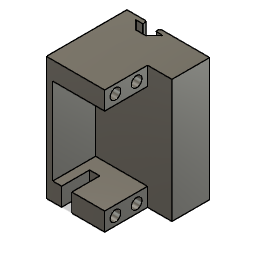
Servo Mount v5 (Autodesk Fusion 360 design; units mm, degrees)
Autodesk Fusion 360 part; units mm, degrees
sketch "Sketch1" plane through (0, 0, 0) normal (0, 0, 1) x (1, 0, 0)
  line L0 (-21, 58) -> (21, 58)
  line L1 (21, 58) -> (21, 0)
  line L2 (21, 0) -> (-21, 0)
  line L3 (-21, 0) -> (-21, 58)
  dimension "d1" = 42
  dimension "d2" = 58
  constraint horizontal L0
  constraint vertical L1
  constraint horizontal L2
  constraint vertical L3
  constraint midpoint origin L2
  measures "d1" distance of L0.start L0.end
  measures "d2" distance of L0.start L2.end
extrude "Extrude1" add sketch "Sketch1" along normal blind 38 makes body 1
sketch "Sketch2" plane through (0, 0, 38) normal (0, 0, 1) x (1, 0, 0)
  line L0 (-21, 0) -> (21, 0)
  line L1 (21, 0) -> (21, 58)
  line L2 (21, 58) -> (-21, 58)
  line L3 (-21, 58) -> (-21, 0)
  line L4 (21, 58) -> (-21, 58)
  line L5 (-21, 58) -> (-21, 0)
  line L6 (-21, 0) -> (21, 0)
  line L7 (21, 0) -> (21, 58)
  line L8 (4, 58) -> (4, 0)
  line L9 (4, 49.4) -> (-18, 49.4)
  line L10 (-18, 49.4) -> (-18, 8.6)
  line L11 (-18, 8.6) -> (4, 8.6)
  line L12 (4, 8.6) -> (4, 49.4)
  line L13 (-18, 49.4) -> (-18, 58) construction
  line L14 (-18, 8.6) -> (-18, 0) construction
  line L15 (-13.8, 8.6) -> (-13.8, 0)
  line L16 (-9, 8.6) -> (-9, 0)
  dimension "d5" = 25
  dimension "d7" = 40.8
  dimension "d8" = 4.2
  dimension "d9" = 4.8
  constraint horizontal L4
  constraint vertical L5
  constraint horizontal L6
  constraint vertical L7
  constraint coincident L0.start L3.end
  constraint coincident L1.end L2.start
  constraint coincident L4 L8.start
  constraint coincident L6 L8.end
  constraint perpendicular L6 L8
  constraint horizontal L9
  constraint vertical L10
  constraint horizontal L11
  constraint vertical L12
  constraint coincident L8 L9.start
  constraint coincident L2 L13.end
  constraint perpendicular L2 L13
  constraint coincident L6 L14.end
  constraint perpendicular L6 L14
  constraint equal L13 L14
  constraint coincident L11 L15.start
  constraint coincident L0 L15.end
  constraint perpendicular L0 L15
  constraint coincident L11 L16.start
  constraint coincident L6 L16.end
  constraint perpendicular L6 L16
  measures "d5" distance of L5 L8
  measures "d7" distance of L9.end L10.end
  measures "d8" distance of L14 L15
  measures "d9" distance of L15 L16
extrude "Extrude2" cut sketch "Sketch2" against normal blind 20.2 contours L8 L9 L10 L11 L12 | L0 L1 L2 L4 L6 L7 L8 L12 bodies 1
extrude "Extrude3" cut sketch "Sketch2" against normal blind 13.2 contours L0 L6 L11 L15 L16 bodies 1
sketch "Sketch3" plane through (0, 58, 0) normal (0, 1, 0) x (-1, 0, 0)
  line L0 (-4, 38) -> (-4, 17.8)
  line L1 (-4, 17.8) -> (-21, 17.8)
  line L2 (-21, 17.8) -> (-21, 0)
  line L3 (-21, 0) -> (21, 0)
  line L4 (21, 0) -> (21, 38)
  line L5 (21, 38) -> (-4, 38)
  line L6 (-21, 0) -> (-18, 0)
  line L7 (-18, 0) -> (-18, 17.8)
  line L8 (-18, 17.8) -> (-21, 17.8)
  line L9 (-21, 17.8) -> (-21, 0)
  dimension "d14" = 3
  constraint horizontal L6
  constraint vertical L7
  constraint horizontal L8
  constraint vertical L9
  constraint coincident L1 L7.end
  constraint coincident L2.end L3.start
  measures "d14" distance of L2.end L6.end
extrude "Extrude4" cut sketch "Sketch3" against normal blind 65 contours L1 L2 L3 L6 L7 L8 L9 bodies 1
sketch "Sketch4" plane through (4, 0, 0) normal (1, 0, 0) x (0, 0, -1)
  line L0 (-38, 58) -> (-38, 49.4)
  line L1 (-38, 49.4) -> (-17.8, 49.4)
  line L2 (-17.8, 49.4) -> (-17.8, 58)
  line L3 (-17.8, 58) -> (-38, 58)
  line L4 (-38, 58) -> (-17.8, 58) construction
  line L5 (-17.8, 58) -> (-17.8, 49.4) construction
  line L6 (-17.8, 49.4) -> (-38, 49.4) construction
  line L7 (-38, 49.4) -> (-38, 58) construction
  line L8 (-27.9, 58) -> (-27.9, 49.4) construction
  line L9 (-38, 53.9) -> (-17.8, 53.9) construction
  line L10 (-32.9, 53.9) -> (-22.9, 53.9)
  circle A0 centre (-32.9, 53.9) radius 2.5
  circle A1 centre (-22.9, 53.9) radius 2.5
  circle A2 centre (-22.9, 4.1) radius 2.5
  line L11 (-22.9, 4.1) -> (-32.9, 4.1) construction
  line L12 (-38, 0) -> (-17.8, 0)
  line L13 (-38, 0) -> (-38, 8.6)
  circle A3 centre (-32.9, 4.1) radius 2.5
  line L14 (-17.8, 0) -> (-38, 0) construction
  line L15 (-17.8, 8.6) -> (-17.8, 0) construction
  line L16 (-27.9, 0) -> (-27.9, 8.6) construction
  line L17 (-17.8, 4.1) -> (-38, 4.1) construction
  line L18 (-17.8, 0) -> (-17.8, 8.6)
  line L19 (-38, 8.6) -> (-38, 0) construction
  line L20 (-17.8, 8.6) -> (-38, 8.6)
  line L21 (-38, 8.6) -> (-17.8, 8.6) construction
  point P0 (-27.9, 53.9)
  point P1 (-27.9, 4.1)
  dimension "d17" = 4.5
  dimension "d18" = 10
  dimension "d19" = 5
  dimension "d20" = 5
  dimension "d21" = 4.5
  dimension "d22" = 10
  dimension "d23" = 5
  dimension "d24" = 5
  constraint horizontal L4
  constraint vertical L5
  constraint horizontal L6
  constraint vertical L7
  constraint coincident L1.end L2.start
  constraint coincident L0.start L3.end
  constraint midpoint L4 L8.start
  constraint midpoint L6 L8.end
  constraint coincident L7 L9.start
  constraint coincident L5 L9.end
  constraint perpendicular L5 L9
  constraint midpoint L9 P0
  constraint coincident L9 L10.start
  constraint coincident L9 L10.end
  constraint parallel L9 L10
  constraint midpoint P0 L10
  constraint coincident L10.start A0.centre
  constraint coincident L10.end A1.centre
  constraint coincident L13.end L19.start
  constraint coincident L12.end L14.start
  constraint midpoint L16.start L14
  constraint midpoint L16.end L21
  constraint coincident L17.start L15
  constraint coincident L17.end L13
  constraint perpendicular L13 L17
  constraint midpoint P1 L17
  constraint coincident A2.centre L17
  constraint coincident L11.end L17
  constraint parallel L11 L17
  constraint midpoint P1 L11
  constraint coincident A2.centre L11.start
  constraint coincident L11.end A3.centre
  measures "d17" distance of L6 L9
  measures "d18" distance of L10.start L10.end
  measures "d19" diameter of A0
  measures "d20" diameter of A1
  measures "d21" distance of L17 L21
  measures "d22" distance of L11.end A2.centre
  measures "d23" diameter of A2
  measures "d24" diameter of A3
extrude "Extrude5" cut sketch "Sketch4" against normal blind 6 contours A0 | A1 | A2 | A3 bodies 1
sketch "profile" plane through (0, 0, 0) normal (0, 1, 0) x (1, 0, 0) in component "20 mm x 20 mm T-Slot v1"
  circle A0 centre (0, 0) radius 2.5
  line L0 (0, -3.9) -> (-2.5, -3.9)
  line L1 (4, -4) -> (-4, 4) construction
  line L2 (-3.9092, -3.9092) -> (4, 4) construction
  line L3 (10, -10) -> (-10, -10) construction
  line L4 (-10, -10) -> (-10, 10) construction
  line L5 (-10, 10) -> (10, 10) construction
  line L6 (10, 10) -> (10, -10) construction
  line L7 (10, -10) -> (-10, 10) construction
  line L8 (-10, -10) -> (10, 10) construction
  line L9 (8, -8) -> (-8, -8) construction
  line L10 (-8, -8) -> (-8, 8) construction
  line L11 (-8, 8) -> (8, 8) construction
  line L12 (8, 8) -> (8, -8) construction
  line L13 (8, -8) -> (-8, 8) construction
  line L14 (-8, -8) -> (8, 8) construction
  line L15 (0, -8) -> (0, -10) construction
  line L16 (0, -9) -> (-3.1, -9) construction
  line L17 (-3.1, -8) -> (-3.1, -9.6)
  line L18 (-1.75, -10) -> (-1.75, -9.6) construction
  line L19 (0, -9.6) -> (-3.5, -9.6) construction
  line L20 (-3.1, -9.6) -> (-3.5, -9.6)
  line L21 (-3.5, -9.6) -> (-3.5, -10)
  line L22 (0, 0) -> (0, -8) construction
  line L23 (-3.5, -10) -> (-10, -10)
  line L24 (-3.9092, -3.9092) -> (-2.5, -3.9) construction
  line L25 (-8, -8) -> (-6.6, -8) construction
  line L26 (-8, -8) -> (-8, -7) construction
  line L27 (-2.5, -3.9) -> (-6.6, -8)
  line L28 (-6.6, -8) -> (-3.1, -8)
  line L29 (0, -2.5) -> (0, -3.9) construction
  line L30 (-3.9, 0) -> (-3.9, -2.5)
  line L31 (-3.9, -2.5) -> (-8, -6.6)
  line L32 (-8, -6.6) -> (-8, -3.1)
  line L33 (-8, -3.1) -> (-9.6, -3.1)
  line L34 (-9.6, -3.1) -> (-9.6, -3.5)
  line L35 (-9.6, -3.5) -> (-10, -3.5)
  line L36 (-10, -3.5) -> (-10, -10)
  line L37 (0, 0) -> (10, 0) construction
  line L38 (3.9, 0) -> (3.9, -2.5)
  line L39 (3.9, -2.5) -> (8, -6.6)
  line L40 (8, -6.6) -> (8, -3.1)
  line L41 (8, -3.1) -> (9.6, -3.1)
  line L42 (9.6, -3.1) -> (9.6, -3.5)
  line L43 (9.6, -3.5) -> (10, -3.5)
  line L44 (10, -3.5) -> (10, -10)
  line L45 (0, -3.9) -> (2.5, -3.9)
  line L46 (6.6, -8) -> (3.1, -8)
  line L47 (3.1, -8) -> (3.1, -9.6)
  line L48 (3.1, -9.6) -> (3.5, -9.6)
  line L49 (3.5, -9.6) -> (3.5, -10)
  line L50 (3.5, -10) -> (10, -10)
  line L51 (2.5, -3.9) -> (6.6, -8)
  line L52 (-3.9, 0) -> (-3.9, 2.5)
  line L53 (-3.9, 2.5) -> (-8, 6.6)
  line L54 (-8, 6.6) -> (-8, 3.1)
  line L55 (-8, 3.1) -> (-9.6, 3.1)
  line L56 (-9.6, 3.1) -> (-9.6, 3.5)
  line L57 (-9.6, 3.5) -> (-10, 3.5)
  line L58 (-10, 3.5) -> (-10, 10)
  line L59 (0, 3.9) -> (-2.5, 3.9)
  line L60 (-6.6, 8) -> (-3.1, 8)
  line L61 (-3.1, 8) -> (-3.1, 9.6)
  line L62 (-3.1, 9.6) -> (-3.5, 9.6)
  line L63 (-3.5, 9.6) -> (-3.5, 10)
  line L64 (-3.5, 10) -> (-10, 10)
  line L65 (-2.5, 3.9) -> (-6.6, 8)
  line L66 (0, 3.9) -> (2.5, 3.9)
  line L67 (6.6, 8) -> (3.1, 8)
  line L68 (3.1, 8) -> (3.1, 9.6)
  line L69 (3.1, 9.6) -> (3.5, 9.6)
  line L70 (3.5, 9.6) -> (3.5, 10)
  line L71 (3.5, 10) -> (10, 10)
  line L72 (2.5, 3.9) -> (6.6, 8)
  line L73 (3.9, 0) -> (3.9, 2.5)
  line L74 (8, 6.6) -> (8, 3.1)
  line L75 (8, 3.1) -> (9.6, 3.1)
  line L76 (9.6, 3.1) -> (9.6, 3.5)
  line L77 (9.6, 3.5) -> (10, 3.5)
  line L78 (10, 3.5) -> (10, 10)
  line L79 (3.9, 2.5) -> (8, 6.6)
  dimension "d3_1" = 5
  dimension "d7_1" = 8
  dimension "d8_1" = 8
  dimension "d9_1" = 20
  dimension "d10_1" = 20
  dimension "d11_1" = 16
  dimension "d12_1" = 16
  dimension "d13_1" = 3.1
  dimension "d14_1" = 0.4
  dimension "d15_1" = 3.5
  dimension "d20_1" = 2.5
  dimension "d21_1" = 1.4
  constraint coincident A0.centre L22.start
  constraint horizontal L0
  constraint coincident L1 A0.centre
  constraint coincident L2 A0.centre
  constraint horizontal L3
  constraint perpendicular L3 L4
  constraint parallel L3 L5
  constraint parallel L4 L6
  constraint coincident L7 A0.centre
  constraint coincident L8 A0.centre
  constraint horizontal L9
  constraint perpendicular L9 L10
  constraint parallel L9 L11
  constraint parallel L10 L12
  constraint coincident L13 A0.centre
  constraint coincident L14 A0.centre
  constraint midpoint L9 L15.start
  constraint midpoint L3 L15.end
  constraint midpoint L15 L16.start
  constraint perpendicular L15 L16
  constraint coincident L9 L17.start
  constraint perpendicular L3 L17
  constraint coincident L16.end L17
  constraint vertical L18
  constraint coincident L3 L18.start
  constraint coincident L15 L19.start
  constraint perpendicular L15 L19
  constraint coincident L18.end L19
  constraint coincident L19 L17.end
  constraint coincident L3 L21.end
  constraint perpendicular L3 L21
  constraint midpoint L18.end L19
  constraint coincident L9 L25.end
  constraint coincident L10 L26.end
  constraint parallel L14 L27
  constraint coincident L22 L0.start
  constraint coincident L22 L29.start
  constraint coincident A0 L29.start
  constraint parallel L22 L29
  constraint coincident L0.start L29.end
  constraint symmetric L3.end L8 L4.start
  constraint symmetric L8 L17.start L32.end
  constraint symmetric L8 L19.end L34.end
  constraint symmetric L8 L17.end L33.end
  constraint symmetric L8 L21.end L35.end
  constraint symmetric L8 L0.end L30.end
  constraint symmetric L8 L25.end L31.end
  constraint symmetric L8 L0.start L30.start
  constraint midpoint L6 L37.end
  constraint symmetric L3.end L22 L3.start
  constraint symmetric L17.start L22 L46.end
  constraint symmetric L19.end L22 L48.end
  constraint symmetric L17.end L22 L47.end
  constraint symmetric L21.end L22 L49.end
  constraint symmetric L22 L0.end L45.end
  constraint symmetric L22 L25.end L46.start
  constraint symmetric L22 L0.start L29.end
  constraint symmetric L22 L30.start L38.start
  constraint symmetric L22 L30.end L38.end
  constraint symmetric L22 L31.end L39.end
  constraint symmetric L22 L32.end L40.end
  constraint symmetric L22 L33.end L41.end
  constraint symmetric L22 L34.end L42.end
  constraint symmetric L22 L35.end L43.end
  constraint symmetric L22 L3.end L3.start
  constraint symmetric L3.end L37 L4.end
  constraint symmetric L17.start L37 L60.end
  constraint symmetric L19.end L37 L62.end
  constraint symmetric L17.end L37 L61.end
  constraint symmetric L21.end L37 L63.end
  constraint symmetric L0.end L37 L59.end
  constraint symmetric L25.end L37 L60.start
  constraint symmetric L0.start L37 L59.start
  constraint symmetric L30.start L37 L52.start
  constraint symmetric L30.end L37 L52.end
  constraint symmetric L31.end L37 L53.end
  constraint symmetric L32.end L37 L54.end
  constraint symmetric L33.end L37 L55.end
  constraint symmetric L34.end L37 L56.end
  constraint symmetric L35.end L37 L57.end
  constraint symmetric L37 L38.start L73.start
  constraint symmetric L37 L38.end L73.end
  constraint symmetric L37 L39.end L74.start
  constraint symmetric L37 L40.end L74.end
  constraint symmetric L37 L41.end L75.end
  constraint symmetric L37 L42.end L76.end
  constraint symmetric L37 L43.end L77.end
  constraint symmetric L37 L3.start L5.end
  constraint symmetric L37 L0.start L59.start
  constraint symmetric L37 L45.end L66.end
  constraint symmetric L37 L46.start L67.start
  constraint symmetric L37 L46.end L67.end
  constraint symmetric L37 L47.end L68.end
  constraint symmetric L37 L48.end L69.end
  constraint symmetric L37 L49.end L70.end
  measures "d3_1" diameter of A0
  measures "d7_1" distance of L1.end L2.end
  measures "d8_1" distance of L1.start L2.end
  measures "d9_1" distance of L4.end L5.end
  measures "d10_1" distance of L3.end L4.end
  measures "d11_1" distance of L10.end L11.end
  measures "d12_1" distance of L9.end L10.end
  measures "d13_1" distance of L16.start L16.end
  measures "d14_1" distance of L18.start L18.end
  measures "d15_1" distance of L19.start L19.end
  measures "d20_1" distance of L0.end L0.start
  measures "d21_1" distance of L29.start L0.start
extrude "Extrude3'" add sketch "profile" along normal blind 10 separate body makes body 2 in component "20 mm x 20 mm T-Slot v1"
fillet "Fillet1" radius 0.6 4 edges at (-10, 5, 10) (10, 5, 10) (10, 5, -10) (-10, 5, -10) on bodies 2 in component "20 mm x 20 mm T-Slot v1"
fillet "Fillet1" radius 0.2 8 edges at (3.1, 5, 8) (8, 5, 3.1) (8, 5, -3.1) (3.1, 5, -8) (-3.1, 5, 8) (-8, 5, 3.1) (-3.1, 5, -8) (-8, 5, -3.1) on bodies 2 in component "20 mm x 20 mm T-Slot v1"
fillet "Fillet1" radius 0.2 8 edges at (-8, 5, 6.6) (-6.6, 5, 8) (6.6, 5, 8) (8, 5, 6.6) (8, 5, -6.6) (6.6, 5, -8) (-6.6, 5, -8) (-8, 5, -6.6) on bodies 2 in component "20 mm x 20 mm T-Slot v1"
fillet "Fillet1" radius 0.4 8 edges at (-2.5, 5, 3.9) (2.5, 5, 3.9) (3.9, 5, 2.5) (3.9, 5, -2.5) (2.5, 5, -3.9) (-2.5, 5, -3.9) (-3.9, 5, -2.5) (-3.9, 5, 2.5) on bodies 2 in component "20 mm x 20 mm T-Slot v1"
sketch "Sketch6" plane through (0, 71, 0) normal (0, 1, 0) x (-1, 0, 0)
  arc A0 (16.7, 6.9) -> (16.5, 6.7) centre (16.7, 6.7) ccw
  line L0 (16.5, 6.7) -> (16.5, 3.8828)
  arc A1 (16.1586, 3.7414) -> (16.5, 3.8828) centre (16.3, 3.8828) ccw
  line L1 (16.1586, 3.7414) -> (12.5172, 7.3828)
  arc A2 (12.4, 7.6657) -> (12.5172, 7.3828) centre (12.8, 7.6657) ccw
  line L2 (12.4, 7.6657) -> (12.4, 12.3343)
  arc A3 (12.5172, 12.6172) -> (12.4, 12.3343) centre (12.8, 12.3343) ccw
  line L3 (12.5172, 12.6172) -> (16.1586, 16.2586)
  arc A4 (16.5, 16.1172) -> (16.1586, 16.2586) centre (16.3, 16.1172) ccw
  line L4 (16.5, 16.1172) -> (16.5, 13.3)
  arc A5 (16.5, 13.3) -> (16.7, 13.1) centre (16.7, 13.3) ccw
  line L5 (16.7, 13.1) -> (18.1, 13.1)
  line L6 (18.1, 13.1) -> (18.1, 13.5)
  line L7 (18.1, 13.5) -> (18.5, 13.5)
  line L8 (18.5, 13.5) -> (18.5, 19.4)
  arc A6 (18.5, 19.4) -> (17.9, 20) centre (17.9, 19.4) ccw
  line L9 (17.9, 20) -> (12, 20)
  line L10 (12, 20) -> (12, 19.6)
  line L11 (12, 19.6) -> (11.6, 19.6)
  line L12 (11.6, 19.6) -> (11.6, 18.2)
  arc A7 (11.6, 18.2) -> (11.8, 18) centre (11.8, 18.2) ccw
  line L13 (11.8, 18) -> (14.6172, 18)
  arc A8 (14.7586, 17.6586) -> (14.6172, 18) centre (14.6172, 17.8) ccw
  line L14 (14.7586, 17.6586) -> (11.1172, 14.0172)
  arc A9 (10.8343, 13.9) -> (11.1172, 14.0172) centre (10.8343, 14.3) ccw
  line L15 (10.8343, 13.9) -> (6.1657, 13.9)
  arc A10 (5.8828, 14.0172) -> (6.1657, 13.9) centre (6.1657, 14.3) ccw
  line L16 (5.8828, 14.0172) -> (2.2414, 17.6586)
  arc A11 (2.3828, 18) -> (2.2414, 17.6586) centre (2.3828, 17.8) ccw
  line L17 (2.3828, 18) -> (5.2, 18)
  arc A12 (5.2, 18) -> (5.4, 18.2) centre (5.2, 18.2) ccw
  line L18 (5.4, 18.2) -> (5.4, 19.6)
  line L19 (5.4, 19.6) -> (5, 19.6)
  line L20 (5, 19.6) -> (5, 20)
  line L21 (5, 20) -> (-0.9, 20)
  arc A13 (-0.9, 20) -> (-1.5, 19.4) centre (-0.9, 19.4) ccw
  line L22 (-1.5, 19.4) -> (-1.5, 13.5)
  line L23 (-1.5, 13.5) -> (-1.1, 13.5)
  line L24 (-1.1, 13.5) -> (-1.1, 13.1)
  line L25 (-1.1, 13.1) -> (0.3, 13.1)
  arc A14 (0.3, 13.1) -> (0.5, 13.3) centre (0.3, 13.3) ccw
  line L26 (0.5, 13.3) -> (0.5, 16.1172)
  arc A15 (0.8414, 16.2586) -> (0.5, 16.1172) centre (0.7, 16.1172) ccw
  line L27 (0.8414, 16.2586) -> (4.4828, 12.6172)
  arc A16 (4.6, 12.3343) -> (4.4828, 12.6172) centre (4.2, 12.3343) ccw
  line L28 (4.6, 12.3343) -> (4.6, 7.6657)
  arc A17 (4.4828, 7.3828) -> (4.6, 7.6657) centre (4.2, 7.6657) ccw
  line L29 (4.4828, 7.3828) -> (0.8414, 3.7414)
  arc A18 (0.5, 3.8828) -> (0.8414, 3.7414) centre (0.7, 3.8828) ccw
  line L30 (0.5, 3.8828) -> (0.5, 6.7)
  arc A19 (0.5, 6.7) -> (0.3, 6.9) centre (0.3, 6.7) ccw
  line L31 (0.3, 6.9) -> (-1.1, 6.9)
  line L32 (-1.1, 6.9) -> (-1.1, 6.5)
  line L33 (-1.1, 6.5) -> (-1.5, 6.5)
  line L34 (-1.5, 6.5) -> (-1.5, 0.6)
  arc A20 (-1.5, 0.6) -> (-0.9, 0) centre (-0.9, 0.6) ccw
  line L35 (-0.9, 0) -> (5, 0)
  line L36 (5, 0) -> (5, 0.4)
  line L37 (5, 0.4) -> (5.4, 0.4)
  line L38 (5.4, 0.4) -> (5.4, 1.8)
  arc A21 (5.4, 1.8) -> (5.2, 2) centre (5.2, 1.8) ccw
  line L39 (5.2, 2) -> (2.3828, 2)
  arc A22 (2.2414, 2.3414) -> (2.3828, 2) centre (2.3828, 2.2) ccw
  line L40 (2.2414, 2.3414) -> (5.8828, 5.9828)
  arc A23 (6.1657, 6.1) -> (5.8828, 5.9828) centre (6.1657, 5.7) ccw
  line L41 (6.1657, 6.1) -> (10.8343, 6.1)
  arc A24 (11.1172, 5.9828) -> (10.8343, 6.1) centre (10.8343, 5.7) ccw
  line L42 (11.1172, 5.9828) -> (14.7586, 2.3414)
  arc A25 (14.6172, 2) -> (14.7586, 2.3414) centre (14.6172, 2.2) ccw
  line L43 (14.6172, 2) -> (11.8, 2)
  arc A26 (11.8, 2) -> (11.6, 1.8) centre (11.8, 1.8) ccw
  line L44 (11.6, 1.8) -> (11.6, 0.4)
  line L45 (11.6, 0.4) -> (12, 0.4)
  line L46 (12, 0.4) -> (12, 0)
  line L47 (12, 0) -> (17.9, 0)
  arc A27 (17.9, 0) -> (18.5, 0.6) centre (17.9, 0.6) ccw
  line L48 (18.5, 0.6) -> (18.5, 6.5)
  line L49 (18.5, 6.5) -> (18.1, 6.5)
  line L50 (18.1, 6.5) -> (18.1, 6.9)
  line L51 (18.1, 6.9) -> (16.7, 6.9)
  circle A28 centre (8.5, 10) radius 2.5
  line L52 (5, 0) -> (12, 0)
  constraint coincident L35.end L36.start
  constraint coincident L46.end L47.start
extrude "Extrude6" cut sketch "Sketch6" against normal blind 75 contours L36 L37 L38 A21 L39 A22 L40 A23 L41 A24 L42 A25 L43 A26 L44 L45 L46 L52 bodies 1
sketch "Sketch1 (2)" plane through (0, 0, 0) normal (0, 0, 1) x (1, 0, 0) in component "Hose Nozzle Holder v3"
  line L0 (0, 25) -> (64, 25)
  line L1 (64, 25) -> (64, -13)
  line L2 (64, -13) -> (0, -13)
  line L3 (0, -13) -> (0, 25)
  dimension "d1_1" = 64
  dimension "d2_1" = 38
  constraint horizontal L0
  constraint vertical L1
  constraint horizontal L2
  constraint vertical L3
  measures "d1_1" distance of L0.start L0.end
  measures "d2_1" distance of L0.start L2.end
extrude "Extrude1'" add sketch "Sketch1 (2)" along normal blind 38 separate body makes body 3 in component "Hose Nozzle Holder v3"
sketch "Sketch2 (2)" plane through (0, 0, 38) normal (0, 0, 1) x (1, 0, 0) in component "Hose Nozzle Holder v3"
  line L0 (0, -13) -> (64, -13)
  line L1 (64, -13) -> (64, 25)
  line L2 (64, 25) -> (0, 25)
  line L3 (0, 25) -> (0, -13)
  line L4 (0, 25) -> (64, -13) construction
  line L5 (40.6603, 21) -> (23.3397, 21)
  line L6 (23.3397, 21) -> (14.6795, 6)
  line L7 (14.6795, 6) -> (23.3397, -9)
  line L8 (23.3397, -9) -> (40.6603, -9)
  line L9 (40.6603, -9) -> (49.3205, 6)
  line L10 (49.3205, 6) -> (40.6603, 21)
  circle A0 centre (32, 6) radius 11.5
  point P0 (32, 6)
  point P1 (32, 6)
  dimension "d5_1" = 15
  dimension "d8_2" = 23
  constraint coincident L2.end L3.start
  constraint coincident L0.end L1.start
  constraint midpoint L4 P1
  constraint coincident P1 P0
  constraint parallel L2 L5
  measures "d5_1" distance of P1 L10
  measures "d8_2" diameter of A0
extrude "Extrude2'" cut sketch "Sketch2 (2)" against normal blind 8 contours L5 L6 L7 L8 L9 L10 | A0 bodies 3 in component "Hose Nozzle Holder v3"
extrude "Extrude3''" cut sketch "Sketch2 (2)" against normal blind 52 contours A0 bodies 3 in component "Hose Nozzle Holder v3"
sketch "Sketch4 (2)" plane through (0, 0, 0) normal (-1, 0, 0) x (0, 0, 1) in component "Hose Nozzle Holder v3"
  line L0 (0, 25) -> (0, -13)
  line L1 (0, -13) -> (38, -13)
  line L2 (38, -13) -> (38, 25)
  line L3 (38, 25) -> (0, 25)
  circle A0 centre (19, 6) radius 6.75 construction
  line L4 (2.0294, 22.9706) -> (35.9706, -10.9706) construction
  line L5 (19, 25) -> (19, -13) construction
  line L6 (2.0294, -10.9706) -> (35.9706, 22.9706) construction
  line L7 (2.0294, 22.9706) -> (11.3071, 6)
  line L8 (2.0294, 22.9706) -> (19, 13.6929)
  line L9 (35.9706, 22.9706) -> (19, 13.6929)
  line L10 (35.9706, 22.9706) -> (26.6929, 6)
  line L11 (35.9706, -10.9706) -> (26.6929, 6)
  line L12 (35.9706, -10.9706) -> (19, -1.6929)
  line L13 (2.0294, -10.9706) -> (19, -1.6929)
  line L14 (2.0294, -10.9706) -> (11.3071, 6)
  line L15 (19, 6) -> (2.0294, 22.9706) construction
  line L16 (8.5702, 16.4298) -> (10.5147, 18.3317) construction
  line L17 (9.9844, 15.0156) -> (12.3158, 17.3471) construction
  line L18 (11.3986, 13.6014) -> (14.1445, 16.3473) construction
  line L19 (12.8128, 12.1872) -> (15.9732, 15.3476) construction
  point P0 (19, 6)
  point P1 (12.8128, 12.1872)
  point P2 (11.3986, 13.6014)
  point P3 (9.9844, 15.0156)
  point P4 (8.5702, 16.4298)
  point P5 (14.227, 10.773)
  dimension "d11_2" = 13.5
  dimension "d12_2" = 48
  dimension "d13_2" = 48
  dimension "d26_1" = 2
  dimension "d27_1" = 2
  dimension "d28_1" = 2
  dimension "d29_1" = 2
  constraint coincident P0 A0.centre
  constraint midpoint L3 L5.start
  constraint midpoint L1 L5.end
  constraint midpoint P0 L5
  constraint midpoint P0 L4
  constraint perpendicular L4 L6
  constraint midpoint P0 L6
  constraint tangent A0 L7
  constraint tangent A0 L8
  constraint tangent A0 L9
  constraint tangent A0 L10
  constraint tangent A0 L11
  constraint tangent A0 L12
  constraint tangent A0 L13
  constraint tangent A0 L14
  constraint coincident L5 L8.end
  constraint coincident L5 L12.end
  constraint coincident L4 P1
  constraint coincident L15 P2
  constraint coincident L15 P3
  constraint coincident L15 P4
  constraint coincident A0 P5
  constraint coincident L4 P5
  constraint coincident P4 L16.start
  constraint midpoint L8 L16.end
  constraint coincident P3 L17.start
  constraint coincident L8 L17.end
  constraint perpendicular L4 L17
  constraint coincident P2 L18.start
  constraint coincident L8 L18.end
  constraint perpendicular L15 L18
  constraint coincident P1 L19.start
  constraint coincident L8 L19.end
  constraint perpendicular L15 L19
  measures "d11_2" diameter of A0
  measures "d12_2" distance of L4.start L4.end
  measures "d13_2" distance of L6.start L6.end
  measures "d26_1" distance of P3 P4
  measures "d27_1" distance of P2 P3
  measures "d28_1" distance of P1 P2
  measures "d29_1" distance of P1 P5
extrude "Extrude4'" cut sketch "Sketch4 (2)" against normal blind 3 contours L7 L8 L9 L10 L11 L12 L13 L14 bodies 3 in component "Hose Nozzle Holder v3"
fillet "Fillet1'" radius 3 2 edges at (32, 25, 0) (32, -13, 0) on bodies 3 in component "Hose Nozzle Holder v3"
fillet "Fillet2" radius 3 2 edges at (32, 25, 38) (32, -13, 38) on bodies 3 in component "Hose Nozzle Holder v3"
sketch "Sketch5" plane through (64, 0, 0) normal (1, 0, 0) x (0, 0, -1) in component "Hose Nozzle Holder v3"
  arc A0 (-38, -10) -> (-35, -13) centre (-35, -10) ccw
  line L0 (-35, -13) -> (-3, -13)
  arc A1 (-3, -13) -> (0, -10) centre (-3, -10) ccw
  line L1 (0, -10) -> (0, 22)
  arc A2 (0, 22) -> (-3, 25) centre (-3, 22) ccw
  line L2 (-3, 25) -> (-35, 25)
  arc A3 (-35, 25) -> (-38, 22) centre (-35, 22) ccw
  line L3 (-38, 22) -> (-38, -10)
  circle A4 centre (-19, 6) radius 11.25
  circle A5 centre (-19, 6) radius 4.5
  point P0 (-19, 25)
  point P1 (-19, -13)
  point P2 (-38, 6)
  point P3 (0, 6)
  point P4 (-19, 6)
  dimension "d20_2" = 22.5
  dimension "d21_2" = 9
  constraint midpoint L2 P0
  constraint midpoint L0 P1
  constraint midpoint L3 P2
  constraint midpoint L1 P3
  constraint coincident P4 A4.centre
  measures "d20_2" diameter of A4
  measures "d21_2" diameter of A5
extrude "Extrude5'" cut sketch "Sketch5" against normal blind 18 contours A5 bodies 3 in component "Hose Nozzle Holder v3"
extrude "Extrude6'" cut sketch "Sketch5" against normal blind 7 contours A4 bodies 3 in component "Hose Nozzle Holder v3"
extrude "Extrude7" add 2 faces at (4, 53.7667, 37.1333) (4, 4.2333, 37.1333) along direction (1, 0, 0) blind 2.5 on bodies 1 bodies 1
sketch "Sketch7" plane through (0, 0, 0) normal (0, -1, 0) x (1, 0, 0)
  line L0 (-12, 0) -> (-12, 0.4)
  line L1 (-12, 0.4) -> (-11.6, 0.4)
  line L2 (-11.6, 0.4) -> (-11.6, 1.8)
  arc A0 (-11.6, 1.8) -> (-11.8, 2) centre (-11.8, 1.8) ccw
  line L3 (-11.8, 2) -> (-14.6172, 2)
  arc A1 (-14.7586, 2.3414) -> (-14.6172, 2) centre (-14.6172, 2.2) ccw
  line L4 (-14.7586, 2.3414) -> (-11.1172, 5.9828)
  arc A2 (-10.8343, 6.1) -> (-11.1172, 5.9828) centre (-10.8343, 5.7) ccw
  line L5 (-10.8343, 6.1) -> (-6.1657, 6.1)
  arc A3 (-5.8828, 5.9828) -> (-6.1657, 6.1) centre (-6.1657, 5.7) ccw
  line L6 (-5.8828, 5.9828) -> (-2.2414, 2.3414)
  arc A4 (-2.3828, 2) -> (-2.2414, 2.3414) centre (-2.3828, 2.2) ccw
  line L7 (-2.3828, 2) -> (-5.2, 2)
  arc A5 (-5.2, 2) -> (-5.4, 1.8) centre (-5.2, 1.8) ccw
  line L8 (-5.4, 1.8) -> (-5.4, 0.4)
  line L9 (-5.4, 0.4) -> (-5, 0.4)
  line L10 (-5, 0.4) -> (-5, 0)
  line L11 (-5, 0) -> (18, 0)
  line L12 (18, 0) -> (18, 17.8)
  line L13 (18, 17.8) -> (6.5, 17.8)
  line L14 (6.5, 17.8) -> (6.5, 38)
  line L15 (6.5, 38) -> (-9, 38)
  line L16 (-9, 38) -> (-9, 24.8)
  line L17 (-9, 24.8) -> (-13.8, 24.8)
  line L18 (-13.8, 24.8) -> (-13.8, 38)
  line L19 (-13.8, 38) -> (-21, 38)
  line L20 (-21, 38) -> (-21, 0)
  line L21 (-21, 0) -> (-12, 0)
  line L22 (-13.8, 24.8) -> (-10.8343, 6.1)
  line L23 (-9, 24.8) -> (-6.1657, 6.1)
  line L24 (-13.8, 24.8) -> (-9, 24.8)
  line L25 (-10.8343, 6.1) -> (-6.1657, 6.1)
  constraint coincident L17.end L18.start
  constraint coincident A2.start L5.start
  constraint coincident L16.end L17.start
  constraint coincident L5.end A3.end
extrude "Extrude8" cut sketch "Sketch7" against normal blind 2 contours L5 L17 L22 L23 L24 L25 bodies 1
component "20 mm x 20 mm T-Slot v1" placed x (1, 0, 0) y (0, 1, 0) z (0, 0, 1) at (-8.5, 61, 10)
component "Hose Nozzle Holder v3" placed x (1, 0, 0) y (0, 1, 0) z (0, 0, 1) at (24.5, 16, 9)
equation "d13_1 = ( 6.2 / 2 ) * 1 mm"
equation "d15_1 = 7 mm / 2"
